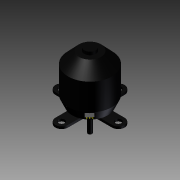
# Autodesk Inventor part: Thrust_Motor
Saved by Autodesk Inventor 2011 SP1 (Build 150282100, 282)
## iProperties
Created: 2011-06-11
Part Number: Thrust_Motor
Document SubType Name: Modeling
Designer: Andrew G. Meyer
Mass: 7.15486 g
Surface Area: 24.3818 cm^2
Volume: 7.15486 cm^3
Density: 1 g/cm^3
Author: Andrew G. Meyer
Autodesk Inventor part; units mm, degrees
ref_plane "YZ Plane" through (0, 0, 0) normal (1, 0, 0) x (0, 1, 0)
ref_plane "XZ Plane" through (0, 0, 0) normal (0, 1, 0) x (-1, 0, 0)
sketch "Sketch1" plane through (0, 0, 0) normal (0, 0, 1) x (1, 0, 0)
  line L0 (-0.9779, 24.003) -> (1.7526, 24.003)
  line L1 (1.7526, 24.003) -> (1.7526, 22.5552)
  line L2 (1.7526, 22.5552) -> (4.2926, 22.5552)
  line L3 (4.2926, 22.5552) -> (9.5377, 17.0688)
  line L4 (9.5377, 17.0688) -> (9.5377, 4.3434)
  line L5 (9.5377, 4.3434) -> (7.5819, 0)
  line L6 (7.5819, 0) -> (0, 0)
  line L7 (-0.9779, -11.5824) -> (-0.9779, 24.003)
  line L8 (-0.9779, -8.6887) -> (-0.9779, -11.5824)
  line L9 (-0.9779, -11.5824) -> (0, -11.5824)
  line L10 (0, -11.5824) -> (0, 0)
  dimension "d0" = 24.003
  dimension "d1" = 10.5156
  dimension "d2" = 22.5552
  dimension "d3" = 17.0688
  dimension "d4" = 4.3434
  dimension "d5" = 2.7305
  dimension "d6" = 11.5824
  dimension "d7" = 0.9779
  dimension "d9" = 5.2705
  dimension "d10" = 8.5598
  constraints: 22 end point, 4 parallel, 3 perpendicular, 1 coincident, 1 collinear, 1 horizontal, 1 point on line
  measures "d0" distance between parallel lines of L6 L0
  measures "d1" distance between parallel lines of L4 L7
  measures "d2" distance between parallel lines of L6 L2
  measures "d3" distance from line of L6 L3.end
  measures "d4" distance from line of L6 L4.end
  measures "d5" distance of L0.start L0.end
  measures "d6" distance of L9.end L6.end
  measures "d7" distance of L7.start L9.end
  measures "d9" distance from line of L2.end L7
  measures "d10" distance from line of L5.end L7
revolve "Revolution1" add sketch "Sketch1" angle 360 about axis through (-0.9779, -11.5824, 0) along (0, 1, 0)
sketch "Sketch2" plane through (-0.9779, 0, 0) normal (0, -1, 0) x (1, 0, 0)
  circle A0 centre (0, 0) radius 0.9779 projected
  circle A1 centre (0, 0) radius 8.5598 projected
  line L0 (6.1849, 3.0099) -> (13.589, 3.0099)
  line L1 (16.5989, 0) -> (16.5989, 0)
  line L2 (13.589, -3.0099) -> (6.1849, -3.0099)
  line L3 (3.0099, -6.1849) -> (3.0099, -13.589)
  line L4 (0, -16.5989) -> (0, -16.5989)
  line L5 (-3.0099, -13.589) -> (-3.0099, -6.1849)
  line L6 (-6.1849, -3.0099) -> (-13.589, -3.0099)
  line L7 (-16.5989, 0) -> (-16.5989, 0)
  line L8 (-13.589, 3.0099) -> (-6.1849, 3.0099)
  line L9 (-3.0099, 6.1849) -> (-3.0099, 13.589)
  line L10 (0, 16.5989) -> (0, 16.5989)
  line L11 (3.0099, 13.589) -> (3.0099, 6.1849)
  arc A2 (-6.1849, 3.0099) -> (-3.0099, 6.1849) centre (-6.1849, 6.1849) ccw
  arc A3 (3.0099, 6.1849) -> (6.1849, 3.0099) centre (6.1849, 6.1849) ccw
  arc A4 (6.1849, -3.0099) -> (3.0099, -6.1849) centre (6.1849, -6.1849) ccw
  arc A5 (-3.0099, -6.1849) -> (-6.1849, -3.0099) centre (-6.1849, -6.1849) ccw
  arc A6 (16.5989, 0) -> (13.589, 3.0099) centre (13.589, 0) ccw
  arc A7 (13.589, -3.0099) -> (16.5989, 0) centre (13.589, 0) ccw
  arc A8 (-13.589, 3.0099) -> (-16.5989, 0) centre (-13.589, 0) ccw
  arc A9 (-16.5989, 0) -> (-13.589, -3.0099) centre (-13.589, 0) ccw
  arc A10 (-3.0099, -13.589) -> (0, -16.5989) centre (0, -13.589) ccw
  arc A11 (0, -16.5989) -> (3.0099, -13.589) centre (0, -13.589) ccw
  arc A12 (0, 16.5989) -> (-3.0099, 13.589) centre (0, 13.589) ccw
  arc A13 (3.0099, 13.589) -> (0, 16.5989) centre (0, 13.589) ccw
  circle A14 centre (0, 0) radius 4.1021
  circle A15 centre (0, 13.589) radius 1.4986
  circle A16 centre (13.589, 0) radius 1.4986
  circle A17 centre (-13.589, 0) radius 1.4986
  circle A18 centre (0, -13.589) radius 1.4986
  point P0 (0.9779, 0)
  dimension "d15" = 6.0198
  dimension "d16" = 3.175
  dimension "d17" = 3.0099
  dimension "d18" = 13.589
  dimension "d19" = 13.589
  dimension "d20" = 13.589
  dimension "d21" = 8.2042
  dimension "d22" = 2.9972
  constraints: 24 end point, 24 point on circle, 24 tangent, 17 centre point, 13 equal radius, 9 parallel, 8 equal length, 5 coincident, 1 collinear, 1 horizontal, 1 horizontal alignment, 1 perpendicular
  measures "d15" distance between parallel lines of L11 L9
  measures "d16" radius of A2
  measures "d17" radius of A6
  measures "d18" distance of point (0, 0) A13.centre
  measures "d19" distance of point (0, 0) A9.centre
  measures "d20" distance of point (0, 0) A10.centre
  measures "d21" diameter of A14
  measures "d22" diameter of A15
extrude "Extrusion1" add sketch "Sketch2" along normal blind 1.0922 contours A1 L2 A4 L3 L5 A5 L6 L8 A2 L9 L11 A3 L0 | A1 L0 A6 A7 L2 | A1 L9 A12 A13 L11 | L3 A11 A10 L5 A1 | A1 L6 A9 A8 L8
ref_plane "Work Plane1" through (5.0748, 0, 6.0527) normal (0.6448, -0.4106, 0.6448) x (0.5371, 0.8435, 0)
sketch "Sketch3" plane through (5.0748, 0, 6.0527) normal (0.6448, -0.4106, 0.6448) x (0.5371, 0.8435, 0)
  line L0 (3.28, 3.0554) -> (4.5151, 0.3869)
  line L1 (2.3848, 2.6411) -> (3.62, -0.0274)
  arc A0 (3.28, 3.0554) -> (2.3848, 2.6411) centre (2.8324, 2.8483) ccw
  arc A1 (3.62, -0.0274) -> (4.5151, 0.3869) centre (4.0675, 0.1797) ccw
  point P0 (-2.7259, -1.8667)
  constraints: 4 end point, 4 point on circle, 3 tangent, 2 centre point, 2 parallel
extrude "Extrusion2" add sketch "Sketch3" along normal blind 1.5875 and the other way blind 0.254
sketch "Sketch4" plane through (6.0983, -0.6518, 7.0762) normal (0.6448, -0.4106, 0.6448) x (0.5438, -0.3463, -0.7644)
  arc A0 (0.0274, 3.62) -> (-0.3869, 4.5151) centre (-0.1797, 4.0675) ccw projected
  arc A1 (-3.0554, 3.28) -> (-2.6411, 2.3848) centre (-2.8483, 2.8324) ccw projected
  line L0 (0.0274, 3.62) -> (-2.6411, 2.3848) projected
  circle A2 centre (-2.4072, 3.0365) radius 0.3811
  circle A3 centre (-1.514, 3.45) radius 0.3811
  circle A4 centre (-0.6208, 3.8634) radius 0.3811
  line L1 (-2.8483, 2.8324) -> (-0.1797, 4.0675) construction
  line L2 (-2.4072, 3.0365) -> (-1.514, 3.45)
  line L3 (-1.514, 3.45) -> (-0.6208, 3.8634)
  line L4 (-2.4072, 3.0365) -> (-2.8483, 2.8324) construction
  line L5 (-2.4072, 3.0365) -> (-2.8483, 2.8324) construction
  line L6 (-0.6208, 3.8634) -> (-0.1797, 4.0675) construction
  point P0 (1.8667, -2.7259)
  constraints: 12 end point, 7 collinear, 3 centre point, 2 equal radius, 2 point on line, 1 midpoint, 1 parallel
extrude "Extrusion3" cut sketch "Sketch4" against normal blind 0.254
sketch "Sketch5" plane through (7.6722, 2.9262, 7.387) normal (0.6448, -0.4106, 0.6448) x (0.7071, 0, -0.7071)
  circle A0 centre (0, 0) radius 0.3811 construction
sketch "Sketch6" plane through (6.9643, 2.8868, 8.0698) normal (0.6448, -0.4106, 0.6448) x (0.7071, 0, -0.7071)
  circle A0 centre (0, 0) radius 0.3811 construction
sketch "Sketch7" plane through (6.2565, 2.8475, 8.7525) normal (0.6448, -0.4106, 0.6448) x (0.7071, 0, -0.7071)
  circle A0 centre (0, 0) radius 0.3811 construction
equation "\"d19\" = d18"
equation "\"d20\" = d18"
body "Solid1"
